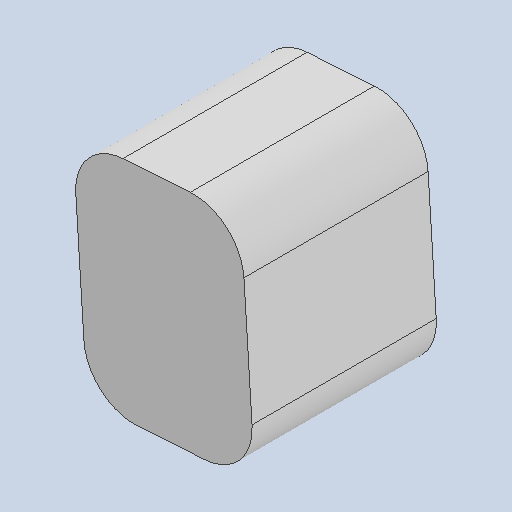
# Autodesk Inventor part: wspornik
Saved by Autodesk Inventor 2022 (Build 260153000, 153)
## iProperties
Created: 2023-01-29
Part Number: wspornik
Material: Generic
Document SubType Name: Modeling
Designer: Kamil
Density: 1 g/cm^3
Appearance: Default
Mass: 37.0634 g
Surface Area: 63.4437 cm^2
Volume: 37.0634 cm^3
Author: Kamil
Autodesk Inventor part; units mm, degrees
ref_plane "YZ Plane" through (0, 0, 0) normal (1, 0, 0) x (0, 1, 0)
ref_plane "XZ Plane" through (0, 0, 0) normal (0, 1, 0) x (-1, 0, 0)
ref_plane "XY Plane" through (0, 0, 0) normal (0, 0, 1) x (1, 0, 0)
sketch "Sketch1" plane through (0, 0, 0) normal (0, 0, 1) x (1, 0, 0)
  circle A0 centre (176.4473, 2.2721) radius 1.6 projected
  arc A1 (177.7566, -17.685) -> (175.138, 22.2292) centre (176.4473, 2.2721) ccw projected
  line L0 (-74.9544, 5.8219) -> (175.138, 22.2292) projected
  line L1 (-72.3358, -34.0923) -> (-74.9544, 5.8219) projected
  line L2 (177.7566, -17.685) -> (-72.3358, -34.0923) projected
  circle A2 centre (176.4473, 2.2721) radius 20
  line L3 (-74.9544, 5.8219) -> (-45.0187, 7.7858)
  line L4 (-45.0187, 7.7858) -> (-42.4001, -32.1284)
  point P0 (0, 0)
  dimension "d0" = 30
  constraints: 4 end point, 2 point on line, 1 centre point, 1 coincident, 1 concentric, 1 perpendicular
  measures "d0" distance of L0.start L3.end
ref_plane "Work Plane1" through (-89.0919, -102.1665, 32.7858) normal (0, 0, -1) x (0, 1, 0)
extrude "Extrusion1" add sketch "Sketch1" along normal up to surface (32.7858 mm away) contours L2 L1 L0 L4
fillet "Fillet1" radius 9 4 edges at (-42.4001, -32.1284, 16.3929) (-72.3358, -34.0923, 16.3929) (-45.0187, 7.7858, 16.3929) (-74.9544, 5.8219, 16.3929)
body "Solid1"
